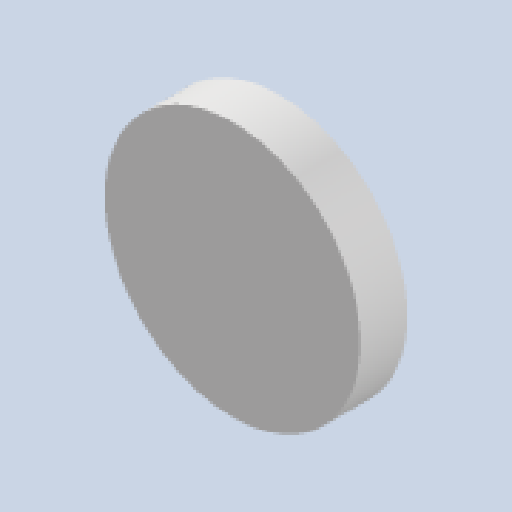
# Autodesk Inventor part: knob
Saved by Autodesk Inventor 2026.2 (Build 302298000, 298)
## iProperties
Created: 2026-04-10
Part Number: knob
Material: Generic
Document SubType Name: Modeling
Designer: Fork
Density: 1 g/cm^3
Appearance: Default
Author: Fork
Autodesk Inventor part; units mm, degrees
ref_plane "YZ Plane" through (0, 0, 0) normal (1, 0, 0) x (0, 1, 0)
ref_plane "XZ Plane" through (0, 0, 0) normal (0, 1, 0) x (-1, 0, 0)
ref_plane "XY Plane" through (0, 0, 0) normal (0, 0, 1) x (1, 0, 0)
sketch "Sketch1" plane through (0, 0, 0) normal (0, 0, 1) x (1, 0, 0)
  circle A0 centre (0.25, 36.05) radius 30
  line L0 (-21, -56.05) -> (-21, -1.05) projected
  line L1 (-21, -1.05) -> (21.5, -1.05) projected
  line L2 (21.5, -1.05) -> (21.5, -56.05) projected
  line L3 (21.5, -56.05) -> (-21, -56.05) projected
  arc A1 (-41, -66.05) -> (-36, -71.05) centre (-36, -66.05) ccw projected
  line L4 (-36, -71.05) -> (36, -71.05) projected
  arc A2 (36, -71.05) -> (41, -66.05) centre (36, -66.05) ccw projected
  line L5 (41, -66.05) -> (41, 71.05) projected
  line L6 (41, 71.05) -> (-41, 71.05) projected
  line L7 (-41, 71.05) -> (-41, -66.05) projected
  circle A3 centre (-36, 66.05) radius 3.25 projected
  circle A4 centre (-36, -66.05) radius 3.25 projected
  circle A5 centre (36, 66.05) radius 3.25 projected
  circle A6 centre (36, -66.05) radius 3.25 projected
  circle A7 centre (0.25, 36.05) radius 3.75 projected
  point P0 (0, 0)
  dimension "d0" = 60
  constraints: 1 centre point
  measures "d0" diameter of A0
extrude "Extrusion1" add sketch "Sketch1" along normal blind 9 contours A0 | A7
sketch "Sketch2" plane through (0.25, 36.05, 0) normal (0, 0, -1) x (-1, 0, 0)
  circle A0 centre (0, 0) radius 3.15
  line L0 (-1.65, 2.6833) -> (-1.65, -2.6833)
  circle A1 centre (0, 0) radius 30 projected
  point P0 (0.25, -36.05)
  dimension "d5" = 6.3
  dimension "d6" = 4.8
  dimension "d7" = 0
  constraints: 2 end point, 2 point on circle, 1 centre point, 1 vertical
  measures "d5" diameter of A0
  measures "d7" distance of A1.centre A0.centre
extrude "Extrusion2" cut sketch "Sketch2" against normal blind 7 contours A0 L0 picked at (1.6001, 0.6823)
sketch "Sketch3" plane through (0.25, 36.05, 0) normal (0, 0, -1) x (-1, 0, 0)
  circle A0 centre (0, 0) radius 3.15
  circle A1 centre (0, 0) radius 7.5
  circle A2 centre (0, 0) radius 25
  circle A3 centre (0, 0) radius 30 projected
  point P0 (0.25, -36.05)
  dimension "d10" = 15
  dimension "d11" = 5
  dimension "d12" = 26.85
  dimension "d13" = 6.3
  constraints: 3 centre point, 2 coincident
  measures "d10" diameter of A1
  measures "d11" radial gap between concentric circles of A3 A2
  measures "d12" radial gap between concentric circles of A3 A0
  measures "d13" diameter of A0
extrude "Extrusion3" cut sketch "Sketch3" against normal blind 7 contours A2
sketch "Sketch4" plane through (0.25, 36.05, 0) normal (0, 0, -1) x (-1, 0, 0)
  circle A0 centre (0, 0) radius 30 projected
  circle A1 centre (0, 0) radius 25 projected
  point P0 (0.25, -36.05)
extrude "Extrusion4" add sketch "Sketch4" along normal blind 6
body "Solid1"
